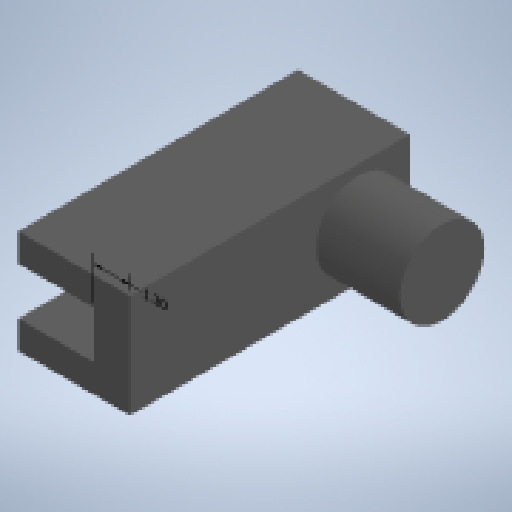
# Autodesk Inventor part: chest_cover_axis_right
Saved by Autodesk Inventor 2024.1 (Build 281209000, 209)
## iProperties
Created: 2024-10-11
Part Number: chest_cover_axis_right
Material: 一般
Document SubType Name: Modeling
Designer: hibik
Density: 1 g/cm^3
Appearance: 既定
Author: hibik
Autodesk Inventor part; units mm, degrees
ref_plane "YZ Plane" through (0, 0, 0) normal (1, 0, 0) x (0, 1, 0)
ref_plane "XZ Plane" through (0, 0, 0) normal (0, 1, 0) x (-1, 0, 0)
ref_plane "XY Plane" through (0, 0, 0) normal (0, 0, 1) x (1, 0, 0)
sketch "スケッチ1" plane through (0, 0, 0) normal (0, 1, 0) x (-1, 0, 0)
  line L0 (0, 0) -> (4, 0)
  line L1 (4, 0) -> (4, 10)
  line L2 (4, 10) -> (0, 10)
  line L3 (0, 10) -> (0, 0)
  dimension "d0" = 4
  dimension "d1" = 10
  constraints: 8 end point, 2 parallel, 1 horizontal, 1 perpendicular
  measures "d0" distance of L2.end L1.end
  measures "d1" distance of L1.end L0.end
extrude "押し出し1" add sketch "スケッチ1" along normal blind 3.7
sketch "スケッチ2" plane through (-4, 0, 10) normal (0, 0, 1) x (1, 0, 0)
  line L0 (0, 0) -> (0, 3.7) projected
  line L1 (0, 2.7) -> (2.7, 2.7)
  line L2 (2.7, 2.7) -> (2.7, 1)
  line L3 (2.7, 1) -> (0, 1)
  line L4 (0, 1) -> (0, 2.7)
  point P0 (4, 0)
  point P1 (0, 1.85)
  dimension "d4" = 2.7
  dimension "d5" = 1.7
  constraints: 8 end point, 2 midpoint, 2 parallel, 1 horizontal, 1 perpendicular, 1 point on line
  measures "d4" distance of L2.end L3.end
  measures "d5" distance of L1.end L2.end
extrude "押し出し2" cut sketch "スケッチ2" against normal through all
sketch "スケッチ3" plane through (0, 0, 10) normal (1, 0, 0) x (0, 0, -1)
  line L0 (0, 0) -> (10, 0) projected
  line L1 (0, 3.7) -> (10, 3.7) projected
  circle A0 centre (8.15, 1.85) radius 1.85
  line L2 (10, 0) -> (10, 3.7) projected
  circle A1 centre (8.15, 1.85) radius 1.5
  dimension "d8" = 3
  constraints: 3 tangent, 2 centre point, 1 coincident
  measures "d8" diameter of A1
extrude "押し出し3" add sketch "スケッチ3" along normal blind 3 contours A1
